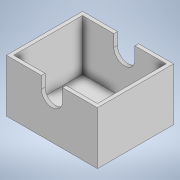
# Autodesk Inventor part: motor_holder#1
Saved by Autodesk Inventor 2021 (Build 250183000, 183)
## iProperties
Created: 2024-03-26
Part Number: motor_holder#1
Material: Generic
Document SubType Name: Modeling
Designer: 23adrdam
Density: 1 g/cm^3
Appearance: Default
Author: 23adrdam
Autodesk Inventor part; units mm, degrees
ref_plane "YZ Plane" through (0, 0, 0) normal (1, 0, 0) x (0, 1, 0)
ref_plane "XZ Plane" through (0, 0, 0) normal (0, 1, 0) x (-1, 0, 0)
ref_plane "XY Plane" through (0, 0, 0) normal (0, 0, 1) x (1, 0, 0)
sketch "Sketch1" plane through (0, 0, 0) normal (0, 1, 0) x (-1, 0, 0)
  line L0 (-11.5, -9.45) -> (11.5, -9.45)
  line L1 (11.5, -9.45) -> (11.5, 9.45)
  line L2 (11.5, 9.45) -> (-11.5, 9.45)
  line L3 (-11.5, 9.45) -> (-11.5, -9.45)
  line L4 (12.5, -10.45) -> (-12.5, -10.45)
  line L5 (-12.5, -10.45) -> (-12.5, 10.45)
  line L6 (-12.5, 10.45) -> (12.5, 10.45)
  line L7 (12.5, 10.45) -> (12.5, -10.45)
  point P0 (0, 0)
  dimension "d0" = 23
  dimension "d4" = 9.45
  dimension "d6" = 11.5
  dimension "d21" = 18.9
  dimension "d22" = 20.9
  dimension "d23" = 10.45
  dimension "d24" = 25
  dimension "d25" = 12.5
  constraints: 16 end point, 4 parallel, 2 horizontal, 2 perpendicular
  measures "d0" distance of L1.end L2.end
  measures "d4" distance from line of point (0, 0) L0
  measures "d6" distance from line of point (0, 0) L3
  measures "d21" distance of L2.end L0.start
  measures "d22" distance of L4.end L5.end
  measures "d23" distance from line of point (0, 0) L6
  measures "d24" distance of L5.end L6.end
  measures "d25" distance from line of point (0, 0) L5
extrude "Extrusion1" add sketch "Sketch1" along normal blind 14
sketch "Sketch2" plane through (0, 0, 0) normal (0, -1, 0) x (1, 0, 0)
  line L0 (2.75, 2.75) -> (-2.75, 2.75)
  line L1 (-2.75, 2.75) -> (-2.75, -2.75)
  line L2 (-2.75, -2.75) -> (2.75, -2.75)
  line L3 (2.75, -2.75) -> (2.75, 2.75)
  line L4 (-12.5, -10.45) -> (-12.5, 10.45) projected
  line L5 (-12.5, 10.45) -> (12.5, 10.45) projected
  line L6 (-12.5, -10.45) -> (-12.5, 10.45) projected
  line L7 (12.5, -10.45) -> (-12.5, -10.45) projected
  line L8 (-12.5, 10.45) -> (12.5, 10.45)
  line L9 (12.5, 10.45) -> (12.5, -10.45)
  line L10 (12.5, -10.45) -> (-12.5, -10.45)
  line L11 (-12.5, -10.45) -> (-12.5, 10.45)
  point P0 (0, 0)
  dimension "d10" = 5.5
  dimension "d11" = 5.5
  dimension "d26" = 2.75
  dimension "d27" = 2.75
  constraints: 16 end point, 4 parallel, 2 horizontal, 2 perpendicular
  measures "d10" distance of L1.end L2.end
  measures "d11" distance of L0.end L1.end
  measures "d26" distance from line of L3 point (0, 0)
  measures "d27" distance from line of L0 point (0, 0)
extrude "Extrusion2" add sketch "Sketch2" along normal blind 0.5
sketch "Sketch4" plane through (-12.5, 14, 10.45) normal (0, 0, 1) x (1, 0, 0)
  line L0 (25, -14.5) -> (0, -14.5) projected
  line L1 (12.5, -14.5) -> (12.5, -3.3) construction
  line L2 (0, 0) -> (0, -14.5) projected
  circle A0 centre (12.5, -3.3) radius 2.9
  line L3 (0, 0) -> (25, 0) projected
  line L4 (12.5, -3.3) -> (15.4, -3.3) construction
  line L5 (12.5, -3.3) -> (9.6, -3.3) construction
  line L6 (15.4, -3.3) -> (15.4, 0)
  line L7 (9.6, -3.3) -> (9.6, 0)
  point P0 (12.5, -14)
  dimension "d28" = 12.5
  dimension "d29" = 11.2
  dimension "d30" = 5.8
  constraints: 10 end point, 2 perpendicular, 2 point on circle, 2 point on line, 2 tangent, 1 centre point, 1 coincident, 1 horizontal, 1 midpoint, 1 vertical
  measures "d28" distance between parallel lines of L2 L1
  measures "d29" distance of L1.start L1.end
  measures "d30" diameter of A0
extrude "Extrusion4" cut sketch "Sketch4" against normal through all
equation "\"d4\" = 0.5 * d1"
equation "\"d6\" = 0.5 * d0"
equation "\"d23\" = 0.5 * d22"
equation "\"d25\" = 0.5 * d24"
equation "\"d11\" = d10"
equation "\"d26\" = 0.5 * d10"
equation "\"d27\" = 0.5 * d11"
equation "\"d1\" = 18.9"
body "Solid1"
